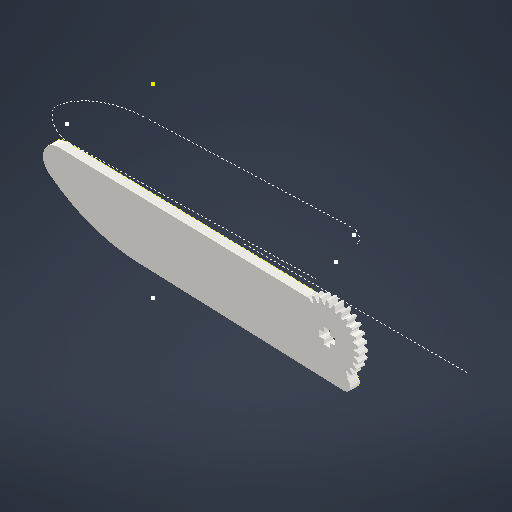
# Autodesk Inventor part: PinzaVieja
Saved by Autodesk Inventor 2026.3 (Build 303398000, 398)
## iProperties
CustomPartVersion: 1
Created: 2026-04-16
Part Number: PinzaVieja
Material: Steel
Document SubType Name: Modeling
Designer: Jose Carlos
Categories: <?xml version="1.0" encoding="UTF-16"?> <MemberInstance><Categories><FamilyTemplate><FamilyTemplateParameter ValueType="xs:double" Id="1" ObjectReferenceKey="da_z" ObjectType="kUserParameterObject"/><FamilyTemplateParameter ValueType="xs:double" Id="2" ObjectReferenceKey="da_b" ObjectType="kUserParameterObject"/><FamilyTemplateParameter ValueType="xs:double" Id="3" ObjectReferenceKey="da_beta" ObjectType="kUserParameterObject"/><FamilyTemplateParameter ValueType="xs:double" Id="4" ObjectReferenceKey="da_da" ObjectType="kUserParameterObject"/><FamilyTemplateParameter ValueType="xs:double" Id="5" ObjectReferenceKey="da_aw" ObjectType="kUserParameterObject"/><FamilyTemplateParameter ValueType="xs:string" Id="6" ObjectReferenceKey="EAIAABAAAACIAQAAAAAAAIAAAAAAAAAA" ObjectType="83910656" SubObjectId="SurfaceGeometry"/></FamilyTemplate><ParamToTemplateMap><ParamToTemplate CategoryParameter="//CategoryParameter[@InternalName='046C89C9-8512-4d59-83FE-43B91F4F132A']" TemplateParameter="1"/><ParamToTemplate CategoryParameter="//CategoryParameter[@InternalName='2552DF32-E462-4b46-AEBF-C6C7768E72AC']" TemplateParameter="2"/><ParamToTemplate CategoryParameter="//CategoryParameter[@InternalName='C9EE641D-15FC-4fae-A226-E94C4372FDD7']" TemplateParameter="3"/><ParamToTemplate><ParamToTemplate CategoryParameter="//CategoryParameter[@InternalName='00B6519A-459B-49c7-AD84-2E56D39A5744']" ConstantValue="0.000000"/></ParamToTemplate><ParamToTemplate><ParamToTemplate CategoryParameter="//CategoryParameter[@InternalName='04B31F0E-C7A6-4894-AA32-9629BEFACF47']" ConstantValue="1.000000"/></ParamToTemplate><ParamToTemplate><ParamToTemplate CategoryParameter="//CategoryParameter[@InternalName='43CBEC2E-7847-49e7-A936-2F7889FCB2D9']" ConstantValue="0.250000"/></ParamToTemplate><ParamToTemplate><ParamToTemplate CategoryParameter="//CategoryParameter[@InternalName='B1EFC894-105D-4ebd-86BF-FA20ED196853']" ConstantValue="0.350000"/></ParamToTemplate><ParamToTemplate><ParamToTemplate CategoryParameter="//CategoryParameter[@InternalName='51175063-3D10-4879-93E8-6246FE8B403D']" ConstantValue="2060000000.000000"/></ParamToTemplate><ParamToTemplate><ParamToTemplate CategoryParameter="//CategoryParameter[@InternalName='A3A52E27-4454-46a9-B0BD-C932399B70AF']" ConstantValue="0.300000"/></ParamToTemplate><ParamToTemplate><ParamToTemplate CategoryParameter="//CategoryParameter[@InternalName='91B76062-C214-41d9-B1B9-14D2AB99603D']" ConstantValue="0.070000"/></ParamToTemplate><ParamToTemplate><ParamToTemplate CategoryParameter="//CategoryParameter[@InternalName='374E806E-8B8A-4dda-A9AA-1039D6500AD2']" ConstantValue="14.285714"/></ParamToTemplate><ParamToTemplate><ParamToTemplate CategoryParameter="//CategoryParameter[@InternalName='2D373A89-B862-43d6-8D0B-0CBF12AB9F6C']" ConstantValue="0.349066"/></ParamToTemplate><ParamToTemplate CategoryParameter="//CategoryParameter[@InternalName='37777632-D6A2-4fac-9D53-DB8ACD95C989']" TemplateParameter="4"/><ParamToTemplate CategoryParameter="//CategoryParameter[@InternalName='FD1017F1-B727-4f7e-9707-0F86F1FF9423']" TemplateParameter="5"/><ParamToTemplate><ParamToTemplate CategoryParameter="//CategoryParameter[@InternalName='9E1B4470-B2D3-4ff1-B813-535BB4CDF51A']" ConstantValue="3520000.000000"/></ParamToTemplate><ParamToTemplate><ParamToTemplate CategoryParameter="//CategoryParameter[@InternalName='F8452263-BFF6-458c-9FB1-07C4B99E95CD']" ConstantValue="11400000.000000"/></ParamToTemplate><ParamToTemplate><ParamToTemplate CategoryParameter="//CategoryParameter[@InternalName='3E3BB259-FD49-497f-8171-6EBC954A3479']" ConstantValue="2.000000"/></ParamToTemplate><ParamToTemplate CategoryParameter="//CategoryParameter[@InternalName='27C3BAF2-7550-4e4b-AE2C-0DB134B7D9B7']" TemplateParameter="6"/></ParamToTemplateMap><Category DisplayName="Gear" InternalName="DC85795E-93AB-48d5-8EEE-5A27447B64BD" Mnemonic="Gear"><CategoryParameter DisplayName="z" InternalName="046C89C9-8512-4d59-83FE-43B91F4F132A" Mnemonic="z"/><CategoryParameter DisplayName="b" InternalName="2552DF32-E462-4b46-AEBF-C6C7768E72AC" Mnemonic="b"/><CategoryParameter DisplayName="||b|" InternalName="C9EE641D-15FC-4fae-A226-E94C4372FDD7" Mnemonic="beta"/><CategoryParameter DisplayName="x" InternalName="00B6519A-459B-49c7-AD84-2E56D39A5744" Mnemonic="x"/><CategoryParameter DisplayName="a*" InternalName="04B31F0E-C7A6-4894-AA32-9629BEFACF47" Mnemonic="a"/><CategoryParameter DisplayName="c*" InternalName="43CBEC2E-7847-49e7-A936-2F7889FCB2D9" Mnemonic="c"/><CategoryParameter DisplayName="r|.f|*" InternalName="B1EFC894-105D-4ebd-86BF-FA20ED196853" Mnemonic="rf"/><CategoryParameter DisplayName="E" InternalName="51175063-3D10-4879-93E8-6246FE8B403D" Mnemonic="E"/><CategoryParameter DisplayName="||m|" InternalName="A3A52E27-4454-46a9-B0BD-C932399B70AF" Mnemonic="mi"/><Category DisplayName="SpurGear" InternalName="26C5A22E-A91E-4dfd-A3B3-23CCAFAE1764" Mnemonic="SpurGear"><CategoryParameter DisplayName="m" InternalName="91B76062-C214-41d9-B1B9-14D2AB99603D" Mnemonic="m"/><CategoryParameter DisplayName="P" InternalName="374E806E-8B8A-4dda-A9AA-1039D6500AD2" Mnemonic="PP"/><CategoryParameter DisplayName="||a|" InternalName="2D373A89-B862-43d6-8D0B-0CBF12AB9F6C" Mnemonic="alpha"/><CategoryParameter DisplayName="d|.a|" InternalName="37777632-D6A2-4fac-9D53-DB8ACD95C989" Mnemonic="da"/><CategoryParameter DisplayName="a|.w|" InternalName="FD1017F1-B727-4f7e-9707-0F86F1FF9423" Mnemonic="aw"/><CategoryParameter DisplayName="||s||.Flim|" InternalName="9E1B4470-B2D3-4ff1-B813-535BB4CDF51A" Mnemonic="sFlim"/><CategoryParameter DisplayName="||s||.Hlim|" InternalName="F8452263-BFF6-458c-9FB1-07C4B99E95CD" Mnemonic="sHlim"/><CategoryParameter DisplayName="tipo" InternalName="3E3BB259-FD49-497f-8171-6EBC954A3479" Mnemonic="type"/><CategoryParameter DisplayName="PitchDiameter" InternalName="27C3BAF2-7550-4e4b-AE2C-0DB134B7D9B7" Mnemonic="IDS_PITCHDIAM"/></Category></Category></Categories></MemberInstance>
Density: 1 g/cm^3
Appearance: Steel
Author: Jose Carlos
Autodesk Inventor part; units mm, degrees
sketch "Sketch1" plane through (0, 0, 0) normal (0, 0, 1) x (1, 0, 0)
  circle A0 centre (0, 0) radius 10.4995
  dimension "d0" = 20.9991
  constraints: 1 centre point
  measures "d0" diameter of A0
extrude "Extrusion1" add sketch "Sketch1" along normal blind 3
ref_plane "Work Plane2" through (0, 0, 1.5) normal (0, 0, 1) x (1, 0, 0)
sketch "Sketch2" plane through (0, 0, 0) normal (0, 0, -1) x (-1, 0, 0)
  circle A0 centre (0, 0) radius 10.4995 projected
  circle A1 centre (0, 0) radius 9.8
  dimension "d3" = 19.6
  constraints: 1 centre point, 1 coincident
  measures "d3" diameter of A1
surface extrude "Diámetro de separación" sketch "Sketch2" against normal through all shown no curves A1
ref_plane "Work Plane8" through (0, 0, 0) normal (0.9937122, 0.1119645, 0) x (0, 0, 1)
ref_plane "Work Plane9" through (0, 0, 0) normal (1, 0, 0) x (0, 1, 0)
spur gear teeth "Engranaje recto" teeth 28 pitch diameter 19.6 tip diameter 20.9991 root diameter 17.85 face width 3 start plane through (0, 0, 0) normal (0, 0, -1) x (-1, 0, 0)
sketch "Boceto3" plane through (0, 0, 0) normal (0, 0, -1) x (-1, 0, 0)
  point P0 (0, 0)
sketch "Boceto4" plane through (0, 0, 0) normal (0, 0, -1) x (-1, 0, 0)
  arc A0 (6.774, 8.022) -> (6.3135, 8.3892) centre (0, 0) ccw construction
  line L0 (6.5464, 8.2089) -> (-6.5464, -8.2089)
  arc A1 (-6.774, -8.022) -> (-6.3135, -8.3892) centre (0, 0) ccw construction
  line L1 (0, 10) -> (100, 10) construction
  line L2 (-43.6, 10) -> (30.6, 10) construction
  line L3 (6.5464, 8.2089) -> (7.9747, 10)
  line L4 (7.9747, 10) -> (100, 10)
  line L5 (100, 10) -> (100, -8.2089)
  line L6 (100, -8.2089) -> (-10, -12.5396)
  line L7 (-10, -12.5396) -> (-6.5464, -8.2089)
  line L8 (0, 0) -> (0, 54.9635) construction
  dimension "d49" = 100
  dimension "d50" = 110
  dimension "d51" = 92.255
  constraints: 18 end point, 5 point on line, 3 point on circle, 2 collinear, 2 horizontal, 2 vertical, 1 midpoint, 2 other
  measures "d49" distance of L1.start L1.end
  measures "d50" horizontal distance of L5.end L6.end
  measures "d51" angle of L5 L6
extrude "Extrusión2" add sketch "Boceto4" against normal up to surface (3 mm away)
fillet "Empalme1" radius 2 1 edges at (10, -12.5396, 1.5)
fillet "Empalme2" radius 50 1 edges at (-100, -8.2089, 1.5)
fillet "Empalme3" radius 5 1 edges at (-100, 10, 1.5)
sketch "Boceto5" plane through (0, 0, 0) normal (0, 0, -1) x (-1, 0, 0)
  arc A0 (91.2606, 1.0819) -> (88.1544, 10) centre (88.1544, 5) ccw construction
  line L0 (7.9747, 10) -> (6.5464, 8.2089) construction
  line L1 (88.1544, 10) -> (6.5464, 8.2089)
  line L2 (88.1544, 10) -> (7.9747, 10) construction
  line L3 (6.5464, 8.2089) -> (7.9747, 10)
  line L4 (7.9747, 10) -> (88.1544, 10)
  point P0 (0, 0)
  constraints: 6 end point, 1 collinear
extrude "Extrusión3" cut sketch "Boceto5" against normal through all
sketch "Boceto6" plane through (0, 0, 0) normal (0, 0, -1) x (-1, 0, 0)
  line L0 (-43.6, 10) -> (30.6, 10) construction
  arc A0 (-7.2747, -9.1222) -> (-5.6324, -12.3676) centre (-5.7111, -10.3692) ccw construction
  line L1 (-6.5464, -8.2089) -> (-7.2747, -9.1222) construction
  line L2 (-5.6324, -12.3676) -> (62.1655, -9.6984) construction
  arc A1 (62.1655, -9.6984) -> (91.2606, 1.0819) centre (60.1985, 40.2629) ccw construction
  arc A2 (91.2606, 1.0819) -> (88.1544, 10) centre (88.1544, 5) ccw construction
  line L3 (88.1544, 10) -> (6.5464, 8.2089) construction
  arc A3 (-5.6324, 32.3676) -> (-7.2747, 29.1222) centre (-5.7111, 30.3692) ccw construction
  line L4 (-6.5464, 28.2089) -> (-7.2747, 29.1222) construction
  line L5 (-5.6324, 32.3676) -> (62.1655, 29.6984) construction
  arc A4 (91.2606, 18.9181) -> (62.1655, 29.6984) centre (60.1985, -20.2629) ccw construction
  arc A5 (88.1544, 10) -> (91.2606, 18.9181) centre (88.1544, 15) ccw construction
  line L6 (88.1544, 10) -> (6.5464, 11.7911) construction
  point P0 (0, 0)
  point P1 (0, 20)
  constraints: 10 symmetric about line, 8 end point, 6 point on circle, 3 centre point, 1 horizontal, 5 other
sketch "Boceto7" plane through (0, 0, 0) normal (0, 0, -1) x (-1, 0, 0)
  line L0 (2.5, -1) -> (-2.5, -1) construction
  line L1 (-2.5, -1) -> (-2.5, 1) construction
  line L2 (-2.5, 1) -> (2.5, 1) construction
  line L3 (2.5, 1) -> (2.5, -1) construction
  line L4 (2.5, -1) -> (-2.5, 1) construction
  line L5 (-2.5, -1) -> (2.5, 1) construction
  line L6 (1, -2.5) -> (-1, -2.5) construction
  line L7 (-1, -2.5) -> (-1, 2.5) construction
  line L8 (-1, 2.5) -> (1, 2.5) construction
  line L9 (1, 2.5) -> (1, -2.5) construction
  line L10 (1, -2.5) -> (-1, 2.5) construction
  line L11 (-1, -2.5) -> (1, 2.5) construction
  line L12 (-1, -1) -> (-2.5, -1)
  line L13 (-2.5, 1) -> (-1, 1)
  line L14 (-2.5, -1) -> (-2.5, 1)
  line L15 (-1, 1) -> (-1, 2.5)
  line L16 (-1, 2.5) -> (1, 2.5)
  line L17 (1, 2.5) -> (1, 1)
  line L18 (1, 1) -> (2.5, 1)
  line L19 (2.5, 1) -> (2.5, -1)
  line L20 (2.5, -1) -> (1, -1)
  line L21 (-1, -2.5) -> (1, -2.5)
  line L22 (1, -1) -> (1, -2.5)
  line L23 (-1, -2.5) -> (-1, -1)
  point P0 (0, 0)
  dimension "d59" = 5
  dimension "d60" = 2
  dimension "d61" = 5
  dimension "d62" = 2
  constraints: 48 end point, 8 point on line, 5 collinear, 5 parallel, 5 perpendicular, 4 midpoint, 2 horizontal
  measures "d59" distance of L0.start L0.end
  measures "d60" distance of L0.end L1.end
  measures "d61" distance of L6.end L7.end
  measures "d62" distance of L6.start L6.end
extrude "Extrusión4" cut sketch "Boceto7" against normal through all
fillet "Empalme4" radius 0.4 4 edges at (1, -1, 1.5) (-1, -1, 1.5) (-1, 1, 1.5) (1, 1, 1.5)
equation "\"d0\" = da_da"
equation "\"d1\" = da_b"
equation "\"d3\" = da_d"
equation "\"da_da\" = 20.999062"
equation "\"da_b\" = 3"
equation "\"da_d\" = 19.6"
body "Solid1"
body "Srf1"
